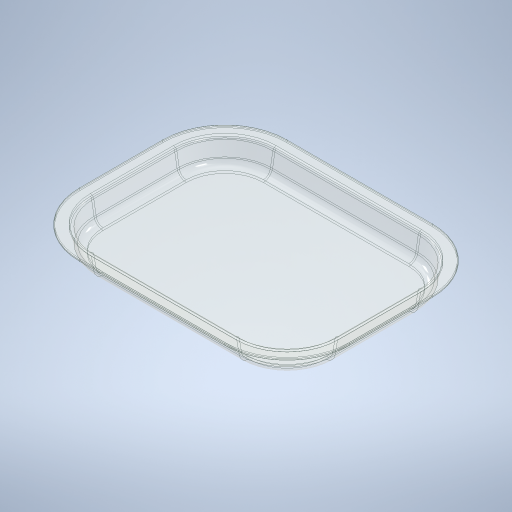
# Autodesk Inventor part: plateau
Saved by Autodesk Inventor 2024 (Build 280153000, 153)
## iProperties
Created: 2024-03-21
Part Number: plateau
Material: Glas
Document SubType Name: Modeling
Designer: ffogue
Density: 2.18 g/cm^3
Appearance: Klar
Author: ffogue
Autodesk Inventor part; units mm, degrees
ref_plane "YZ Plane" through (0, 0, 0) normal (1, 0, 0) x (0, 1, 0)
ref_plane "XZ Plane" through (0, 0, 0) normal (0, 1, 0) x (-1, 0, 0)
ref_plane "XY Plane" through (0, 0, 0) normal (0, 0, 1) x (1, 0, 0)
sketch "Skizze1" plane through (0, 0, 0) normal (0, 0, 1) x (1, 0, 0)
  line L0 (-175, -130) -> (175, -130)
  line L1 (175, -130) -> (175, 130)
  line L2 (175, 130) -> (-175, 130)
  line L3 (-175, 130) -> (-175, -130)
  line L4 (-175, -130) -> (175, 130) construction
  line L5 (175, -130) -> (-175, 130) construction
  point P0 (0, 0)
  dimension "d0" = 350
  dimension "d1" = 260
  constraints: 12 end point, 2 midpoint, 2 parallel, 1 horizontal, 1 perpendicular
  measures "d0" distance of L2.end L1.end
  measures "d1" distance of L1.end L0.end
extrude "Extrusion1" add sketch "Skizze1" along normal blind 33.5
fillet "Rundung1" radius 70 4 edges at (-175, -130, 16.75) (-175, 130, 16.75) (175, 130, 16.75) (175, -130, 16.75)
draft "Flächenverjüngung1" angle -10 pull direction (0, 0, 1) faces at (-35, -130, 11.1667) (112.317, -129.6165, 11.1667) (-159.4002, -104.0524, 11.1667) (175, -20, 22.3333) (-175, 20, 22.3333) (174.9041, 63.6635, 11.1667) (-143.1247, 118.7069, 11.1667) (35, 130, 11.1667) fixed edges at (0, -130, 33.5) (154.4975, -109.4975, 33.5) (-154.4975, -109.4975, 33.5) (175, 0, 33.5) (-175, 0, 33.5) (154.4975, 109.4975, 33.5) (-154.4975, 109.4975, 33.5) (0, 130, 33.5)
fillet "Rundung2" radius 10 8 edges at (0, -124.093, 0) (150.3206, -105.3206, 0) (169.093, 0, 0) (150.3206, 105.3206, 0) (0, 124.093, 0) (-150.3206, 105.3206, 0) (-169.093, 0, 0) (-150.3206, -105.3206, 0)
shell "Wandung1" thickness 3.5 outward yes removed faces 1 at (35, -43.3333, 33.5)
sketch "Skizze2" plane through (0, 0, 0) normal (0, 1, 0) x (-1, 0, 0)
  line L0 (175, 33.5) -> (195, 33.5)
  line L1 (195, 33.5) -> (195, 30)
  line L2 (195, 30) -> (175, 30)
  line L3 (175, 30) -> (175, 33.5)
  point P0 (0, 0)
  dimension "d8" = 20
  dimension "d9" = 3.5
  constraints: 8 end point, 2 parallel, 1 horizontal, 1 perpendicular
  measures "d8" distance of L1.end L2.end
  measures "d9" distance of L0.end L1.end
sketch3d "3D-Skizze1"
  line L0 (-178.554, 60, 33.5) -> (-178.554, -60, 33.5)
  arc A0 (-178.554, -60, 33.5) -> (-105, -133.554, 33.5) centre (-105, -60, 33.5) ccw
  line L1 (-105, -133.554, 33.5) -> (105, -133.554, 33.5)
  arc A1 (105, -133.554, 33.5) -> (178.554, -60, 33.5) centre (105, -60, 33.5) ccw
  line L2 (178.554, -60, 33.5) -> (178.554, 60, 33.5)
  arc A2 (178.554, 60, 33.5) -> (105, 133.554, 33.5) centre (105, 60, 33.5) ccw
  line L3 (105, 133.554, 33.5) -> (-105, 133.554, 33.5)
  arc A3 (-105, 133.554, 33.5) -> (-178.554, 60, 33.5) centre (-105, 60, 33.5) ccw
sweep "Sweeping1" add profiles "Skizze2" path "3D-Skizze1"
fillet "Rundung3" radius 5 8 edges at (-154.4975, 109.4975, 33.5) (0, 130, 33.5) (154.4975, 109.4975, 33.5) (175, 0, 33.5) (154.4975, -109.4975, 33.5) (0, -130, 33.5) (-154.4975, -109.4975, 33.5) (-175, 0, 33.5)
fillet "Rundung4" radius 1.5 8 edges at (-177.9368, 0, 30) (-156.5741, 111.5741, 30) (0, 132.9368, 30) (156.5741, 111.5741, 30) (177.9368, 0, 30) (156.5741, -111.5741, 30) (0, -132.9368, 30) (-156.5741, -111.5741, 30)
fillet "Rundung5" radius 1 16 edges at (0, -150, 30) (168.6396, -123.6396, 30) (195, 0, 30) (168.6396, 123.6396, 30) (0, 150, 30) (-168.6396, 123.6396, 30) (-195, 0, 30) (-168.6396, -123.6396, 30) (0, -150, 33.5) (168.6396, -123.6396, 33.5) (195, 0, 33.5) (168.6396, 123.6396, 33.5) (0, 150, 33.5) (-168.6396, 123.6396, 33.5) (-195, 0, 33.5) (-168.6396, -123.6396, 33.5)
sketch "Skizze3" plane through (-105, -115.702, 0) normal (-1, 0, 0) x (0, 0, 1)
  line L0 (33.5, -18.4934) -> (33.5, -33.298) projected
  arc A0 (33.5, -18.4934) -> (29.3682, -13.5694) centre (28.5, -18.4934) ccw projected
  line L1 (8.2635, -9.8481) -> (29.3682, -13.5694) projected
  arc A1 (0, 0) -> (8.2635, -9.8481) centre (10, 0) ccw projected
  line L2 (0, 55.702) -> (0, 0) projected
  line L3 (-3.5, 55.702) -> (0, 55.702) projected
  line L4 (-3.5, 0) -> (-3.5, 55.702) projected
  arc A2 (-3.5, 0) -> (7.6557, -13.2949) centre (10, 0) ccw projected
  line L5 (7.6557, -13.2949) -> (28.7605, -17.0162) projected
  arc A3 (30, -18.4934) -> (28.7605, -17.0162) centre (28.5, -18.4934) ccw projected
  line L6 (30, -33.298) -> (30, -18.4934) projected
  arc A4 (30, -33.298) -> (31, -34.298) centre (31, -33.298) ccw projected
  line L7 (32.5, -34.298) -> (31, -34.298) projected
  arc A5 (32.5, -34.298) -> (33.5, -33.298) centre (32.5, -33.298) ccw projected
  point P0 (0, 115.702)
